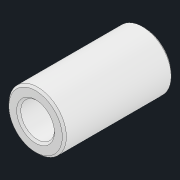
# Autodesk Inventor part: spacer11
Saved by Autodesk Inventor 2021 (Build 250183000, 183)
## iProperties
Created: 2021-07-17
Part Number: spacer11
Material: ABS プラスチック
Document SubType Name: Modeling
Designer: yuta0
Density: 1.06 g/cm^3
Appearance: 滑らか - 白
購入先: 印刷
在庫数: 0.0
Author: yuta0
Autodesk Inventor part; units mm, degrees
ref_plane "YZ Plane" through (0, 0, 0) normal (1, 0, 0) x (0, 1, 0)
ref_plane "XZ Plane" through (0, 0, 0) normal (0, 1, 0) x (-1, 0, 0)
ref_plane "XY Plane" through (0, 0, 0) normal (0, 0, 1) x (1, 0, 0)
sketch "スケッチ1" plane through (0, 0, 0) normal (0, 0, 1) x (1, 0, 0)
  circle A0 centre (0, 0) radius 4.1
  circle A1 centre (0, 0) radius 7
  dimension "d0" = 8.2
  dimension "d1" = 14
  constraints: 2 centre point, 2 coincident
  measures "d0" diameter of A0
  measures "d1" diameter of A1
extrude "押し出し1" add sketch "スケッチ1" along normal mid plane 26.5
chamfer "面取り1" distance 0.5 angle 45 4 edges at (-7, 0, 13.25) (-4.1, 0, 13.25) (-7, 0, -13.25) (-4.1, 0, -13.25)
